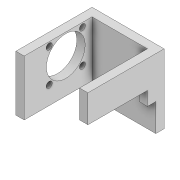
# Autodesk Inventor part: Print_Parts_H1
Saved by Autodesk Inventor 2020.1 (Build 241239000, 239)
## iProperties
Created: 2020-10-29
Part Number: Print_Parts_H1
Material: 一般
Document SubType Name: Modeling
Designer: kenta iguchi
Density: 1 g/cm^3
Appearance: 既定
Author: kenta iguchi
Autodesk Inventor part; units mm, degrees
ref_plane "YZ Plane" through (0, 0, 0) normal (1, 0, 0) x (0, 1, 0)
ref_plane "XZ Plane" through (0, 0, 0) normal (0, 1, 0) x (-1, 0, 0)
ref_plane "XY Plane" through (0, 0, 0) normal (0, 0, 1) x (1, 0, 0)
sketch "スケッチ1" plane through (0, 0, 0) normal (0, 0, 1) x (1, 0, 0)
  circle A0 centre (0, 0) radius 14
  line L0 (-12, -12) -> (12, -12)
  line L1 (12, -12) -> (12, 12)
  line L2 (12, 12) -> (-12, 12)
  line L3 (-12, 12) -> (-12, -12)
  line L4 (-12, -12) -> (12, 12) construction
  line L5 (12, -12) -> (-12, 12) construction
  circle A1 centre (-12, 12) radius 1.45
  circle A2 centre (12, 12) radius 1.45
  circle A3 centre (-12, -12) radius 1.45
  circle A4 centre (12, -12) radius 1.45
  line L6 (-20, -15) -> (20, -15)
  line L7 (20, -15) -> (20, 15)
  line L8 (20, 15) -> (-20, 15)
  line L9 (-20, 15) -> (-20, -15)
  line L10 (-20, -15) -> (20, 15) construction
  line L11 (20, -15) -> (-20, 15) construction
  dimension "d0" = 24
  dimension "d1" = 24
  dimension "d2" = 28
  dimension "d3" = 2.9
  dimension "d4" = 2.9
  dimension "d5" = 2.9
  dimension "d6" = 2.9
  dimension "d7" = 30
  dimension "d8" = 40
  constraints: 24 end point, 5 centre point, 5 coincident, 4 midpoint, 4 parallel, 2 horizontal, 2 perpendicular
  measures "d0" distance of L2.end L1.end
  measures "d1" distance of L1.end L0.end
  measures "d2" diameter of A0
  measures "d3" diameter of A1
  measures "d4" diameter of A2
  measures "d5" diameter of A3
  measures "d6" diameter of A4
  measures "d7" distance of L6.end L7.end
  measures "d8" distance of L7.end L8.end
extrude "押し出し1" add sketch "スケッチ1" along normal blind 6 contours A0 L1 | L1 A0 L0 L3 L2 | A0 L2 A2 L1 | L1 A4 L0 A0 | L2 A0 | A2 L2 L1 | L1 L2 A2 | A0 L0 | A4 L0 L1 | L1 L0 A4 | A0 L3 A1 L2 | L0 A3 L3 A0 | L3 A0 | A1 L3 L2 | L2 L3 A1 | A3 L3 L0 | L0 L3 A3 | L9 L8 L7 L6
sketch "スケッチ3" plane through (0, 0, 0) normal (0, 0, -1) x (-1, 0, 0)
  line L0 (-20, -15) -> (-20, 15) projected
  line L1 (20, 15) -> (20, -15) projected
  line L2 (-20, 15) -> (-26, 15)
  line L3 (-26, 15) -> (-26, -15)
  line L4 (-26, -15) -> (-20, -15)
  line L5 (-20, -15) -> (-20, 15)
  line L6 (20, -15) -> (26, -15)
  line L7 (26, -15) -> (26, 15)
  line L8 (26, 15) -> (20, 15)
  line L9 (20, 15) -> (20, -15)
  dimension "d16" = 6
  dimension "d17" = 6
  constraints: 16 end point, 4 parallel, 3 horizontal alignment, 2 horizontal, 2 perpendicular
  measures "d16" distance of L0.end L2.end
  measures "d17" distance of L7.end L8.end
extrude "押し出し2" add sketch "スケッチ3" against normal blind 55
sketch "スケッチ7" plane through (-26, -15, 0) normal (0, -1, 0) x (1, 0, 0)
  line L0 (52, 0) -> (0, 0) projected
  line L1 (52, 0) -> (52, 55) projected
  line L2 (6, 6) -> (46, 6) projected
  line L3 (0, 0) -> (0, 55) projected
  line L4 (52, 0) -> (0, 0) projected
  line L5 (0, 0) -> (52, 0)
  line L6 (52, 0) -> (52, 6)
  line L7 (52, 6) -> (0, 6)
  line L8 (0, 6) -> (0, 0)
  point P0 (26, 0)
  point P1 (0, 6)
  constraints: 8 end point, 2 parallel, 1 horizontal, 1 horizontal alignment, 1 perpendicular, 1 point on line
extrude "押し出し5" add sketch "スケッチ7" along normal blind 20
sketch "スケッチ8" plane through (0, 0, 0) normal (0, 0, -1) x (-1, 0, 0)
  line L0 (-26, 15) -> (26, 15) projected
  line L1 (26, -35) -> (26, 15) projected
  circle A0 centre (-1.5, -10.4) radius 25.65
  circle A1 centre (21.5, -30.4) radius 1.6
  circle A2 centre (-21.5, 7.6) radius 1.6
  point P0 (0, 0)
  dimension "d29" = 51.3
  dimension "d30" = 3.2
  dimension "d31" = 3.2
  dimension "d34" = 20
  dimension "d35" = 18
  dimension "d36" = 23
  dimension "d37" = 20
  dimension "d38" = 45.4
  dimension "d39" = 4.5
  constraints: 3 centre point
  measures "d29" diameter of A0
  measures "d30" diameter of A1
  measures "d31" diameter of A2
  measures "d34" horizontal distance of A2.centre A0.centre
  measures "d35" vertical distance of A0.centre A2.centre
  measures "d36" horizontal distance of A0.centre A1.centre
  measures "d37" vertical distance of A1.centre A0.centre
  measures "d38" distance from line of A1.centre L0
  measures "d39" distance from line of A1.centre L1
hole "穴1" at (-21.5, -30.4, 0) at (21.5, 7.6, 0) direction (0, 0, 1) diameter 4.4 depth 5
sketch "Sketch10" plane through (-26, -15, 55) normal (-1, 0, 0) x (0, 0, 1)
  line L0 (-55, -20) -> (-55, 30) projected
  line L1 (-49, -20) -> (-55, -20) projected
  line L2 (-49, 0) -> (-49, -20) projected
  line L3 (-49, 0) -> (0, 0) projected
  line L4 (0, 30) -> (0, 0) projected
  line L5 (-55, 30) -> (0, 30) projected
  circle A0 centre (-30, 15) radius 14
  point P0 (-55, 15)
  dimension "d58" = 28
  dimension "d59" = 15
  dimension "d60" = 25
  constraints: 1 centre point
  measures "d58" diameter of A0
  measures "d59" distance from line of A0.centre L3
  measures "d60" distance from line of A0.centre L0
extrude "Extrusion7" cut sketch "Sketch10" against normal blind 10 contours A0
sketch "Sketch11" plane through (-26, -15, 55) normal (-1, 0, 0) x (0, 0, 1)
  circle A0 centre (-30, 15) radius 14 projected
  line L0 (-18, 27) -> (-42, 27)
  line L1 (-42, 27) -> (-42, 3)
  line L2 (-42, 3) -> (-18, 3)
  line L3 (-18, 3) -> (-18, 27)
  line L4 (-18, 27) -> (-42, 3) construction
  line L5 (-42, 27) -> (-18, 3) construction
  point P0 (-55, 15)
  dimension "d63" = 24
  dimension "d64" = 24
  constraints: 12 end point, 2 midpoint, 2 parallel, 1 horizontal, 1 perpendicular
  measures "d63" distance of L2.end L1.end
  measures "d64" distance of L1.end L0.end
hole "Hole2" at (-26, -12, 37) at (-26, 12, 37) at (-26, 12, 13) at (-26, -12, 13) direction (1, 0, 0) diameter 4.4 depth 8.8 tip angle 118
sketch "スケッチ12" plane through (26, -15, 55) normal (1, 0, 0) x (0, 0, -1)
  line L0 (0, 0) -> (0, 30) projected
  line L1 (49, 0) -> (0, 0) projected
  line L2 (49, 0) -> (49, -20) projected
  line L3 (49, 0) -> (0, 0) projected
  line L4 (0, 0) -> (43, 0)
  line L5 (43, 0) -> (43, 10)
  line L6 (43, 10) -> (0, 10)
  line L7 (0, 10) -> (0, 0)
  point P0 (55, 15)
  point P1 (0, 10)
  dimension "d75" = 10
  dimension "d76" = 6
  constraints: 8 end point, 2 parallel, 1 horizontal, 1 perpendicular
  measures "d75" distance of L4.end L5.end
  measures "d76" distance between parallel lines of L5 L2
extrude "押し出し8" cut sketch "スケッチ12" against normal blind 10
sketch "スケッチ13" plane through (-26, -15, 6) normal (0, -1, 0) x (1, 0, 0)
  line L0 (0, 0) -> (6, 0) projected
  line L1 (6, 0) -> (6, 49) projected
  line L2 (0, 49) -> (6, 49) projected
  line L3 (0, 0) -> (0, 49) projected
  point P0 (26, -6)
extrude "押し出し9" add sketch "スケッチ13" along normal blind 10
